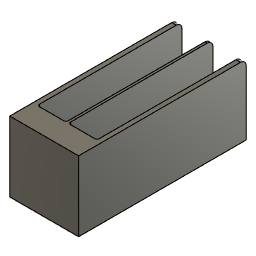
Support Batterie v4 (Autodesk Fusion 360 design; units mm, degrees)
Autodesk Fusion 360 part; units mm, degrees
sketch "Sketch1" plane through (0, 0, 0) normal (0, 1, 0) x (1, 0, 0)
  line L0 (-30, 73) -> (30, 73)
  line L1 (30, 73) -> (30, -73)
  line L2 (30, -73) -> (-30, -73)
  line L3 (-30, -73) -> (-30, 73)
  line L4 (-26, 69) -> (-1, 69)
  line L5 (-1, 69) -> (-1, -69)
  line L6 (-1, -69) -> (-26, -69)
  line L7 (-26, -69) -> (-26, 69)
  line L8 (-26, 69) -> (26, 69)
  line L9 (26, 69) -> (26, -69)
  line L10 (26, -69) -> (-26, -69)
  line L11 (-26, -69) -> (-26, 69)
  line L12 (30, -73) -> (-30, 73) construction
  line L13 (26, 69) -> (1, 69)
  line L14 (1, 69) -> (1, -69)
  line L15 (26, -64) -> (26, 69)
  line L16 (-26, 69) -> (-26, 73)
  line L17 (26, 69) -> (26, 73)
  line L18 (-1, 69) -> (-1, 73)
  line L19 (1, 69) -> (1, 73)
  dimension "d1" = 60
  dimension "d2" = 146
  dimension "d3" = 25
  dimension "d4" = 138
  dimension "d5" = 4
  dimension "d6" = 25
  dimension "d7" = 133
  constraint horizontal L0
  constraint vertical L1
  constraint horizontal L2
  constraint vertical L3
  constraint horizontal L4
  constraint vertical L5
  constraint horizontal L6
  constraint vertical L7
  constraint midpoint origin L12
  constraint horizontal L13
  constraint vertical L14
  constraint vertical L15
  constraint coincident L0 L16.end
  constraint perpendicular L0 L16
  constraint coincident L0 L17.end
  constraint perpendicular L0 L17
  constraint coincident L0 L18.end
  constraint perpendicular L0 L18
  constraint coincident L0 L19.end
  constraint perpendicular L0 L19
  constraint coincident L10 L14.end
  measures "d1" distance of L0.start L0.end
  measures "d2" distance of L0.start L2.end
  measures "d3" distance of L4.end L4.start
  measures "d4" distance of L6.end L4.start
  measures "d6" distance of L8.end L13.end
  measures "d7" distance of L8.end L15.start
extrude "Extrude1" add sketch "Sketch1" along normal blind 49 contours L0 L1 L2 L3 L6 L7 L9 L10 L11 L15 L16 L17 | L0 L8 L18 L19 | L5 L8 L10 L14
extrude "Extrude2" add sketch "Sketch1" against normal blind 10
extrude "Extrude3" add sketch "Sketch1" along normal blind 15 contours L0 L4 L8 L16 L18 | L0 L8 L13 L17 L19
sketch "Sketch2" plane through (0, 49, 0) normal (0, 1, 0) x (-1, 0, 0)
  line L0 (-1, 69) -> (-1, -73)
  line L1 (-1, -73) -> (1, -73)
  line L2 (1, -73) -> (1, 69)
  line L3 (1, 69) -> (26, 69)
  line L4 (26, 69) -> (26, -73)
  line L5 (26, -73) -> (30, -73)
  line L6 (30, -73) -> (30, 73)
  line L7 (30, 73) -> (-30, 73)
  line L8 (-30, 73) -> (-30, -73)
  line L9 (-30, -73) -> (-26, -73)
  line L10 (-26, -73) -> (-26, 69)
  line L11 (-26, 69) -> (-1, 69)
  line L12 (30, 73) -> (-30, 73)
  line L13 (-30, 73) -> (-30, 53)
  line L14 (-30, 53) -> (30, 53)
  line L15 (30, 53) -> (30, 73)
  dimension "d14" = 20
  constraint horizontal L12
  constraint vertical L13
  constraint horizontal L14
  constraint vertical L15
  constraint coincident L6.end L7.start
  measures "d14" distance of L6.end L14.end
extrude "Extrude4" add sketch "Sketch2" along normal blind 2 contours L0 L2 L3 L4 L6 L7 L8 L10 L11 L12 L13 L14 L15 | L0 L10 L11 L14 | L2 L3 L4 L14
extrude "Extrude5" add 3 faces at (28.6667, 49, 11) (0.3333, 49, -31) (-27.3333, 49, -31) along direction (0, 1, 0) blind 2
fillet "Fillet1" radius 5 3 edges at (28, 51, -73) (0, 51, -73) (-28, 51, -73)
fillet "Fillet2" radius 2 4 edges at (1, 50, 53) (-26, 50, 53) (-1, 50, 53) (26, 50, 53)
sketch "Sketch3" plane through (0, 0, 0) normal (0, 1, 0) x (-1, 0, 0)
  line L0 (1, -69) -> (26, -69)
  line L1 (26, -69) -> (26, 69)
  line L2 (26, 69) -> (1, 69)
  line L3 (1, 69) -> (1, -69)
  circle A0 centre (13.5, -50) radius 2.25
  circle A1 centre (13.5, 50) radius 2.25
  line L4 (13.5, -50) -> (13.5, 50)
  line L5 (26, 0) -> (1, 0)
  dimension "d24" = 4.5
  dimension "d26" = 4.5
  dimension "d43" = 100
  constraint coincident A0.centre L4.start
  constraint coincident A1.centre L4.end
  constraint vertical L4
  constraint midpoint L1 L5.start
  constraint midpoint L3 L5.end
  constraint midpoint L4 L5
  measures "d24" diameter of A0
  measures "d26" diameter of A1
  measures "d43" distance of A0.centre A1.centre
extrude "Extrude6" cut sketch "Sketch3" against normal blind 10 contours A0 | A1
sketch "Sketch4" plane through (0, 0, 0) normal (0, 1, 0) x (-1, 0, 0)
  circle A0 centre (13.5, -50) radius 2.25
  circle A1 centre (13.5, 50) radius 2.25
  line L0 (1, -69) -> (26, -69)
  line L1 (26, -69) -> (26, 69)
  line L2 (26, 69) -> (1, 69)
  line L3 (1, 69) -> (1, -69)
  circle A2 centre (13.5, -50) radius 5
  circle A3 centre (13.5, 50) radius 5
  dimension "d29" = 10
  dimension "d30" = 10
  constraint concentric A0 A2
  constraint concentric A1 A3
  measures "d29" diameter of A2
  measures "d30" diameter of A3
extrude "Extrude7" cut sketch "Sketch4" against normal blind 5 contours A2 | A3
sketch "Sketch5" plane through (0, 0, 0) normal (0, 1, 0) x (-1, 0, 0)
  line L0 (-26, -69) -> (-1, -69)
  line L1 (-1, -69) -> (-1, 69)
  line L2 (-1, 69) -> (-26, 69)
  line L3 (-26, 69) -> (-26, -69)
  circle A0 centre (-13.5, -50) radius 2.25
  circle A1 centre (-13.5, 50) radius 2.25
  circle A2 centre (-13.5, -50) radius 5
  circle A3 centre (-13.5, 50) radius 5
  line L4 (-13.5, 50) -> (-13.5, -50)
  line L5 (-1, 0) -> (-26, 0)
  dimension "d35" = 4.5
  dimension "d36" = 4.5
  dimension "d37" = 10
  dimension "d38" = 10
  dimension "d44" = 100
  constraint concentric A0 A2
  constraint concentric A1 A3
  constraint coincident A1.centre A3.centre
  constraint coincident A0.centre A2.centre
  constraint vertical L4
  constraint midpoint L1 L5.start
  constraint midpoint L3 L5.end
  constraint midpoint L4 L5
  measures "d35" diameter of A0
  measures "d36" diameter of A1
  measures "d37" diameter of A2
  measures "d38" diameter of A3
  measures "d44" distance of A1.centre A0.centre
extrude "Extrude8" cut sketch "Sketch5" against normal blind 10 contours A0 | A1
extrude "Extrude9" cut sketch "Sketch5" against normal blind 5 contours A2 | A3
equation "d1 = ( 25 * 2 ) * 1 mm + 10 mm"
equation "d2 = 138 mm + 8 mm"
named bodies: "SuppotBatterie"
